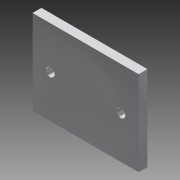
# Autodesk Inventor part: Plate
Saved by Autodesk Inventor 2013 (Build 170138000, 138)
## iProperties
Created: 2014-07-18
Part Number: Plate
Material: Aluminum 6061
Document SubType Name: Modeling
Designer: Kyle
Density: 1 g/cm^3
Author: Kyle
Autodesk Inventor part; units mm, degrees
ref_plane "YZ Plane" through (0, 0, 0) normal (1, 0, 0) x (0, 1, 0)
ref_plane "XZ Plane" through (0, 0, 0) normal (0, 1, 0) x (-1, 0, 0)
ref_plane "XY Plane" through (0, 0, 0) normal (0, 0, 1) x (1, 0, 0)
sketch "Sketch1" plane through (0, 0, 0) normal (0, 0, 1) x (1, 0, 0)
  line L0 (0, 0) -> (38.1, 0)
  line L1 (38.1, 0) -> (38.1, -30.48)
  line L2 (38.1, -30.48) -> (0, -30.48)
  line L3 (0, -30.48) -> (0, 0)
  circle A0 centre (6.35, -15.24) radius 1.5875
  circle A1 centre (31.75, -15.24) radius 1.5875
  dimension "d0" = 38.1
  dimension "d1" = 30.48
  dimension "d2" = 6.35
  dimension "d3" = 6.35
  dimension "d4" = 3.175
  dimension "d5" = 3.175
  constraints: 8 end point, 2 centre point, 2 parallel, 1 horizontal, 1 perpendicular
  measures "d0" distance of L0.start L0.end
  measures "d1" distance of L2.end L0.start
  measures "d2" distance from line of L3 A0.centre
  measures "d3" distance from line of L1 A1.centre
  measures "d4" diameter of A1
  measures "d5" diameter of A0
extrude "Extrusion1" add sketch "Sketch1" along normal blind 3.175
body "Solid1"
